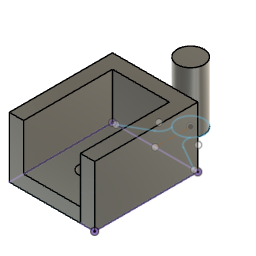
VI Hook v1.0 (Autodesk Fusion 360 design; units mm, degrees)
Autodesk Fusion 360 part; units mm, degrees
note: some values were not read from the file. Set by a fixed rule: which sketch regions a step uses.
sketch "Sketch4" plane through (0, 0, 0) normal (0, 0, 1) x (1, 0, 0)
  circle A0 centre (0, 0) radius 2.5
  line L0 (0, 0) -> (0, 5) construction
  circle A1 centre (0, -10) radius 2.5
  line L1 (0, 5) -> (0, -20) construction
  line L2 (0, -20) -> (-8, -20)
  line L3 (0, -20) -> (8, -20)
  line L4 (0, 5) -> (8, 5)
  line L5 (0, 5) -> (-8, 5)
  line L6 (-8, 5) -> (-8, -20)
  line L7 (8, -20) -> (8, 5)
  line L8 (-8, -20) -> (-12, -20)
  line L9 (-12, -20) -> (-12, 9)
  line L10 (-12, 9) -> (12, 9)
  line L11 (12, 9) -> (12, -20)
  line L12 (12, -20) -> (8, -20)
  dimension "d31" = 5
  dimension "d32" = 5
  dimension "d35" = 0
  dimension "d36" = -10
  dimension "d38" = 8
  dimension "d39" = 8
  dimension "d58" = 8
  dimension "d59" = 8
  dimension "d60" = 4
  dimension "d61" = 29
  dimension "d62" = 24
  constraint coincident A0.centre L0.start
  constraint vertical L0
  constraint parallel L0 L1
  constraint perpendicular L1 L2
  constraint perpendicular L1 L3
  constraint perpendicular L1 L4
  constraint perpendicular L0 L5
  constraint perpendicular L6 L8
  constraint perpendicular L8 L9
  constraint perpendicular L9 L10
  constraint perpendicular L10 L11
  measures "d31" diameter of A0
  measures "d32" distance of A0.centre L0.end
  measures "d38" distance of L1.end L2.end
  measures "d39" distance of L1.end L3.end
  measures "d58" distance of L0.end L4.end
  measures "d59" distance of L0.end L5.end
  measures "d60" distance of L2.end L8.end
  measures "d61" distance of L8.end L9.end
  measures "d62" distance of L9.end L10.end
extrude "Extrude7" add sketch "Sketch4" along normal blind 4 contours L2 L3 L4 L5 L6 L7 makes body 1
extrude "Extrude8" add sketch "Sketch4" along normal blind 17 contours L4 L5 L6 L7 L8 L9 L10 L11 L12 bodies 1
sketch "Sketch5" plane through (0, 0, 0) normal (0, 0, -1) x (1, 0, 0)
  circle A0 centre (0, 0) radius 2.5
  circle A1 centre (0, 10) radius 2.5
  line L0 (8, 20) -> (-12, 20)
  line L1 (0, -9) -> (0, -19) construction
  circle A2 centre (0, -19) radius 3.75
  line L2 (11, -9) -> (4.0043, -12.9748)
  line L3 (-4.0043, -12.9748) -> (-11, -9)
  arc A3 (4.0043, -12.9748) -> (2.5646, -16.2641) centre (5.4863, -15.5832) ccw
  arc A4 (-2.5646, -16.2641) -> (-4.0043, -12.9748) centre (-5.4863, -15.5832) ccw
  line L4 (-12, 20) -> (-12, -9)
  line L5 (-12, -9) -> (12, -9)
  line L6 (12, -9) -> (12, 20)
  line L7 (12, 20) -> (8, 20)
  dimension "d48" = 7.5
  dimension "d49" = 3
  constraint coincident L1.end A2.centre
  constraint tangent L2 A3
  constraint tangent L3 A4
  constraint equal A3 A4
  constraint coincident A2 A3.end
  constraint coincident A2 A4.start
  measures "d48" diameter of A2
  measures "d49" radius of A3
extrude "Extrude9" add sketch "Sketch5" against normal blind 5 separate body contours A2 L2 L3 A3 A4 L5 makes body 2
extrude "Extrude10" add sketch "Sketch5" against normal blind 17 contours A2 bodies 2
fillet "Fillet4" radius 1 tangency weight 2 1 edges at (-2.5646, 16.2641, 2.5) on bodies 2
fillet "Fillet5" radius 1 1 edges at (2.5646, 16.2641, 2.5) on bodies 2
